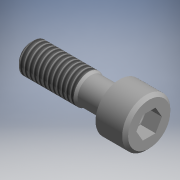
# Autodesk Inventor part: HCBST8-24_Screw
Saved by Autodesk Inventor 2017.3 (Build 213256000, 256)
## iProperties
Part Number: HCBST8-24_Screw
Material: Generic
Catalog Web Link: www.cadenas.de
Description: HCBSTscrew-Frame Washer Assembled Hexagon Socket Head Cap Screws for Aluminum Frames
Vendor: MISUMI
Document SubType Name: Modeling
Designer: partserver
Manufacturer: MISUMI
Mass: 2.03358 g
Surface Area: 12.4304 cm^2
Volume: 2.03358 cm^3
Density: 1 g/cm^3
Appearance: PSOLRGB-192-192-192
Category: PARTsolutions
Company: MISUMI
Title: HCBST8-24_Screw
Author: Cadenas PARTsolutions
Comments: Frame Washer Assembled Hexagon Socket Head Cap Screws for Aluminum Frames
PSOL_IDENT_0: {$CADENAS_DATA\23d-libs\misumi\metric\38_al_extrusions_blackets\nuts\hcbst_screw.prj},177 {VTYP=3D},
PSOL_IDENT_1: {NB=HCBST8-24_Screw},{LINA=HCBST8-24_Screw},{NN=HCBSTscrew},{DATE=17.06.2021 07:12:01},{GEOMDATE=15.
PSOL_IDENT_2: 04.2019 02:00:05},{VERSION=},{LINEID=110},{WBVAR=L},{WBNUMERIC=L}  {NB=HCBST8-24_Screw},{LINA=HCBST8
PSOL_IDENT_3: -24_Screw},{KT=DUMMY},{PN=HCBST8-24_Screw},{TYPE=HCBST},{MATB=Structural Alloy Steel},{HARD=32~44HRC
PSOL_IDENT_4: },{MATSW=JIS B1251},{MATFW=JIS B1256},{ST=Trivalent Chromate},{M=8},{L=24},{M1=8.000},{L0=20,24,29},
PSOL_IDENT_5: {NDM=8},{KDM=6.464163},{MP=8X1.25},{P=1.25},{A=13.0},{E=8},{B=6},{C=14.5},{D=17.0},{AA=8.4}
NB: HCBST8-24_Screw
NN: HCBSTscrew
NT: Frame Washer Assembled Hexagon Socket Head Cap Screws for Aluminum Frames
NBSYN: $PN.
LINA: HCBST8-24_Screw
CATALOG: Misumi
PN: HCBST8-24_Screw
MATB: Structural Alloy Steel
HARD: 32~44HRC
MATSW: JIS B1251
MATFW: JIS B1256
ST: Trivalent Chromate
M: 8
L: 24
MP: 8X1.25
A: 13
E: 8
B: 6
C: 14.5
D: 17
AA: 8.4
SUPPLIER: MISUMI
ARTICLENO: HCBST8-24_Screw
BOMINFO: HCBST8-24_Screw
CREATOR: CADENAS GmbH
Autodesk Inventor part; units mm, degrees
sketch "Sketch_6" plane through (0, 0, 0) normal (0, 0, 1) x (1, 0, 0)
  line L0 (24, 0) -> (7.0715, 0)
  line L1 (7.0715, 0) -> (7.0715, 3.233)
  line L2 (7.0715, 3.233) -> (8.4, 4)
  line L3 (8.4, 4) -> (23.233, 4)
  line L4 (23.233, 4) -> (24, 3.233)
  line L5 (24, 3.233) -> (24, 0)
  line L6 (24, 0) -> (7.0715, 0)
  constraints: 14 end point
revolve "Revolution1" add sketch "Sketch_6" angle 360 about axis through (24, 0, 0) along (1, 0, 0)
thread "Thread1" size "M8x1.25" class "6g" standard "ISO Metric profile" full length
sketch "Sketch_1" plane through (0, 0, 0) normal (0, 0, 1) x (1, 0, 0)
  line L0 (8.4, 0) -> (-8, 0)
  line L1 (-2.2679, 0) -> (-4, 3)
  line L2 (-4, 3) -> (-8, 3)
  line L3 (-8, 3) -> (-8, 5.7)
  line L4 (-8, 5.7) -> (-7.2, 6.5)
  line L5 (-7.2, 6.5) -> (0, 6.5)
  line L6 (0, 6.5) -> (0, 3.616)
  line L7 (0, 3.616) -> (8.4, 3.616)
  line L8 (8.4, 3.616) -> (8.4, 0)
  line L9 (8.4, 0) -> (-2.2679, 0)
  constraints: 20 end point
revolve "Revolution2" add sketch "Sketch_1" angle 360 about axis through (8.4, 0, 0) along (1, 0, 0)
sketch "Sketch_2" plane through (-8, 0, 0) normal (1, 0, 0) x (0, 0, -1)
  line L0 (-3, -1.7321) -> (0, -3.4641)
  line L1 (0, -3.4641) -> (3, -1.7321)
  line L2 (3, -1.7321) -> (3, 1.7321)
  line L3 (3, 1.7321) -> (0, 3.4641)
  line L4 (0, 3.4641) -> (-3, 1.7321)
  line L5 (-3, 1.7321) -> (-3, -1.7321)
  constraints: 12 end point
extrude "Extrusion1" cut sketch "Sketch_2" along normal blind 4
ref_plane "bolt_to_plane_washer_XY" through (5.6, 0, 0) normal (1, 0, 0) x (0, 0, -1)
ref_plane "bolt_to_plane_washer_YZ" through (5.6, 0, 0) normal (0, 0, -1) x (0, 1, 0)
ref_plane "bolt_to_plane_washer_ZX" through (5.6, 0, 0) normal (0, 1, 0) x (1, 0, 0)
ref_plane "bolt_to_spring_washer_XY" through (2.8, 0, 0) normal (1, 0, 0) x (0, 0, -1)
ref_plane "bolt_to_spring_washer_YZ" through (2.8, 0, 0) normal (0, 0, -1) x (0, 1, 0)
ref_plane "bolt_to_spring_washer_ZX" through (2.8, 0, 0) normal (0, 1, 0) x (1, 0, 0)
ref_plane "screw_to_body_XY" through (0, 0, 0) normal (1, 0, 0) x (0, 0, -1)
ref_plane "screw_to_body_YZ" through (0, 0, 0) normal (0, 0, -1) x (0, 1, 0)
ref_plane "screw_to_body_ZX" through (0, 0, 0) normal (0, 1, 0) x (1, 0, 0)
ref_plane "to_washer_XY" through (24, 0, 0) normal (1, 0, 0) x (0, 0, -1)
ref_plane "to_washer_YZ" through (24, 0, 0) normal (0, 0, -1) x (0, 1, 0)
ref_plane "to_washer_ZX" through (24, 0, 0) normal (0, 1, 0) x (1, 0, 0)
body "Solid1"
